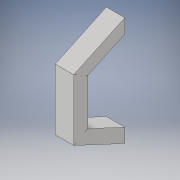
# Autodesk Inventor part: FrameMainMotorMount
Saved by Autodesk Inventor 2019 (Build 230136000, 136)
## iProperties
Created: 2018-08-17
Part Number: FrameMainMotorMount
Material: Generic
Document SubType Name: Modeling
Designer: Kitte_X
Density: 1 g/cm^3
Appearance: Default
Author: Kitte_X
Autodesk Inventor part; units mm, degrees
ref_plane "YZ Plane" through (0, 0, 0) normal (1, 0, 0) x (0, 1, 0)
ref_plane "XZ Plane" through (0, 0, 0) normal (0, 1, 0) x (-1, 0, 0)
ref_plane "XY Plane" through (0, 0, 0) normal (0, 0, 1) x (1, 0, 0)
sketch "Sketch1" plane through (0, 0, 0) normal (1, 0, 0) x (0, 1, 0)
  line L0 (109, 0) -> (-109, 0) construction
  line L1 (147, 0) -> (-147, 0) construction
  line L2 (109, 0) -> (215.066, 0) construction
  line L3 (109, 0) -> (62.3692, 100)
  line L4 (109, 0) -> (219.3378, 0) construction
  line L5 (-147, 0) -> (3, 0) construction
  line L6 (-109, 0) -> (-62.3692, 100)
  line L7 (-109, 0) -> (1.3378, 0) construction
  line L8 (147, 0) -> (82.6495, 138)
  line L9 (82.6495, 138) -> (-82.6495, 138)
  line L10 (-82.6495, 138) -> (-147, 0)
  line L11 (62.3692, 100) -> (-62.3692, 100)
  line L12 (147, 0) -> (109, 0)
  line L13 (-109, 0) -> (-147, 0)
  line L14 (-62.3692, 100) -> (-82.6495, 138) construction
  line L15 (62.3338, 100) -> (82.6141, 138)
  line L16 (82.6661, 137.9646) -> (62.3858, 99.9646)
  line L17 (62.3692, 100) -> (82.6495, 138) construction
  line L18 (-62.3338, 100) -> (-82.6141, 138)
  line L19 (-82.6661, 137.9646) -> (-62.3858, 99.9646)
  point P0 (0, 0)
  point P1 (0, 0)
  point P2 (0, 0)
  dimension "d0" = 218
  dimension "d1" = 294
  dimension "d5" = 115
  dimension "d9" = 65
  dimension "d10" = 38
  dimension "d11" = 100
  dimension "d12" = 0.0625
  dimension "d13" = 0.0625
  dimension "d14" = 0.0312
  dimension "d15" = 0.0312
  constraints: 40 end point, 9 point on line, 7 horizontal, 6 parallel, 3 coincident, 3 collinear, 2 equal length, 2 midpoint
  measures "d0" distance of L0.start L0.end
  measures "d1" distance of L1.start L1.end
  measures "d5" angle of L4 L3
  measures "d9" angle of L7 L6
  measures "d10" distance between parallel lines of L9 L11
  measures "d11" vertical distance of L0.start L3.end
  measures "d12" distance between parallel lines of L16 L15
  measures "d13" distance between parallel lines of L18 L19
  measures "d14" distance between parallel lines of L19 L14
  measures "d15" distance between parallel lines of L16 L17
extrude "Extrusion1" add sketch "Sketch1" along normal blind 50 contours L3 L16 L8 L12 | L11 L18 L9 L15 | L6 L13 L10 L19
sketch "Sketch2" plane through (50, 0, 0) normal (1, 0, 0) x (0, 0, -1)
  line L0 (0, 109) -> (0, 147) construction
  line L1 (0, 147) -> (-137.9646, 82.6661) construction
  line L2 (-137.9646, 82.6661) -> (-99.9646, 62.3858) construction
  line L3 (-99.9646, 62.3858) -> (0, 109) construction
  line L4 (-100, 62.3338) -> (-138, 82.6141) construction
  line L5 (-138, 82.6141) -> (-138, -82.6141) construction
  line L6 (-138, -82.6141) -> (-100, -62.3338) construction
  line L7 (-100, -62.3338) -> (-100, 62.3338) construction
  line L8 (0, -109) -> (-99.9646, -62.3858) construction
  line L9 (-99.9646, -62.3858) -> (-137.9646, -82.6661) construction
  line L10 (-137.9646, -82.6661) -> (0, -147) construction
  line L11 (0, -147) -> (0, -109) construction
  line L12 (0, 109) -> (-100, 62.3692) construction
  line L13 (-100, 62.3692) -> (-100, -62.3692) construction
  line L14 (0, -109) -> (-99.9646, -62.3858) construction
  line L15 (-100, -62.3692) -> (0, -109) construction
  line L16 (0, -147) -> (0, -109) construction
  line L17 (0, -109) -> (0, -147) construction
  line L18 (0, -147) -> (-138, -82.6495) construction
  line L19 (-137.9646, -82.6661) -> (0, -147) construction
  line L20 (-138, -82.6495) -> (-138, 82.6495) construction
  line L21 (0, 109) -> (0, 147) construction
  line L22 (-138, 82.6495) -> (0, 147) construction
  line L23 (0, 147) -> (0, 109) construction
  line L24 (-106.5, 66.5102) -> (0, 116.172)
  line L25 (0, 139.828) -> (-131.5, 78.5086)
  line L26 (-131.5, 78.5086) -> (-131.5, -78.5086)
  line L27 (-131.5, -78.5086) -> (0, -139.828)
  line L28 (0, -116.172) -> (-106.5, -66.5102)
  line L29 (-106.5, -66.5102) -> (-106.5, 66.5102)
  line L30 (0, -147) -> (0, -109) projected
  line L31 (0, 139.828) -> (0, 116.172)
  line L32 (0, -116.172) -> (0, -139.828)
  point P0 (0, 0)
  dimension "d18" = 6.5
  constraints: 32 end point, 8 point on line, 6 collinear, 2 parallel, 3 other
  measures "d18" distance between parallel lines of L12 L24
extrude "Extrusion2" cut sketch "Sketch2" against normal blind 43.5
extrude "Extrusion3" add sketch "Sketch2" against normal blind 6.5
body "Solid1"
